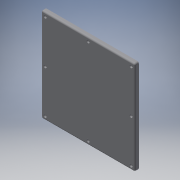
# Autodesk Inventor part: raspberry_box_lid
Saved by Autodesk Inventor 2019 (Build 230136000, 136)
## iProperties
Created: 2022-12-05
Part Number: raspberry_box_lid
Material: S235JR
Document SubType Name: Modellieren
Designer: Damiano Pezzè
Density: 1 g/cm^3
Appearance: Vorgabe
Author: Damiano Pezzè
Autodesk Inventor part; units mm, degrees
ref_plane "YZ Ebene" through (0, 0, 0) normal (1, 0, 0) x (0, 1, 0)
ref_plane "XZ Ebene" through (0, 0, 0) normal (0, 1, 0) x (-1, 0, 0)
ref_plane "XY Ebene" through (0, 0, 0) normal (0, 0, 1) x (1, 0, 0)
sketch "Sketch20" plane through (0, 0, 0) normal (0, 1, 0) x (-1, 0, 0)
  line L0 (0, 0) -> (120, 0)
  line L1 (120, 0) -> (120, -120)
  line L2 (120, -120) -> (0, -120)
  line L3 (0, -120) -> (0, 0)
  dimension "d58" = 120
  dimension "d59" = 120
  constraints: 8 end point, 2 parallel, 1 horizontal, 1 perpendicular
  measures "d58" distance of L1.end L2.end
  measures "d59" distance of L0.end L1.end
extrude "Extrusion8" add sketch "Sketch20" against normal blind 5
fillet "Fillet5" radius 2 8 edges at (-60, -5, 0) (0, -2.5, 0) (0, -5, -60) (0, -2.5, -120) (-60, -5, -120) (-120, -5, -60) (-120, -2.5, -120) (-120, -2.5, 0)
sketch "Sketch21" plane through (0, -5, 0) normal (0, -1, 0) x (1, 0, 0)
  line L0 (-2, 0) -> (-118, 0) projected
  line L1 (0, -118) -> (0, -2) projected
  line L2 (-120, -2) -> (-120, -118) projected
  line L3 (-118, -120) -> (-2, -120) projected
  point P0 (0, 0)
  point P1 (-5, -5)
  point P2 (-60, -5)
  point P3 (-115, -5)
  point P4 (-115, -5)
  point P5 (-115, -115)
  point P6 (-5, -115)
  point P7 (-5, -60)
  point P8 (-115, -60)
  point P9 (-60, -115)
  dimension "d63" = 5
  dimension "d64" = 5
  dimension "d65" = 55
  dimension "d66" = 5
  dimension "d67" = 5
  dimension "d68" = 55
  dimension "d69" = 5
  dimension "d70" = 5
  dimension "d71" = 55
  constraints: 1 coincident
  measures "d63" distance from line of L0 point (-5, -5)
  measures "d64" distance from line of L1 point (-5, -5)
  measures "d65" distance of point (-5, -5) point (-60, -5)
  measures "d66" distance from line of L0 point (-115, -5)
  measures "d67" distance from line of point (-115, -5) L2
  measures "d68" distance of point (-60, -5) point (-115, -5)
  measures "d69" distance from line of L3 point (-115, -115)
  measures "d70" distance from line of L3 point (-60, -115)
  measures "d71" distance of point (-5, -115) point (-60, -115)
hole "Hole2" at (-5, -5, -5) at (-60, -5, -5) at (-115, -5, -5) at (-115, -5, -115) at (-5, -5, -115) at (-5, -5, -60) at (-115, -5, -60) at (-60, -5, -115) direction (0, 1, 0) diameter 2.46 depth 8.8 counterbore diameter 4 counterbore depth 2 thread size "M3x0.5" class "6H" standard "ISO Metric profile"
body "Solid1"
